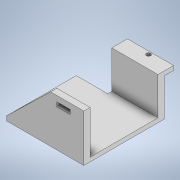
# Autodesk Inventor part: tray2
Saved by Autodesk Inventor 2020 (Build 240168000, 168)
## iProperties
Created: 2022-07-19
Part Number: tray2
Material: 일반
Document SubType Name: Modeling
Designer: SeungJin
Density: 1 g/cm^3
Appearance: 기본값
Author: SeungJin
Autodesk Inventor part; units mm, degrees
ref_plane "YZ Plane" through (0, 0, 0) normal (1, 0, 0) x (0, 1, 0)
ref_plane "XZ Plane" through (0, 0, 0) normal (0, 1, 0) x (-1, 0, 0)
ref_plane "XY Plane" through (0, 0, 0) normal (0, 0, 1) x (1, 0, 0)
sketch "스케치1" plane through (0, 0, 0) normal (0, 1, 0) x (-1, 0, 0)
  line L0 (70.5, 0) -> (70.5, 50)
  line L1 (70.5, 50) -> (0, 50)
  line L2 (0, 50) -> (0, 0)
  line L3 (24.5, 227.5) -> (-40, 227.5)
  line L4 (10, 242.5) -> (37.5, 242.5)
  line L5 (10, 227.5) -> (10, 242.5)
  line L6 (145.5, 227.5) -> (85.5, 227.5)
  line L7 (145.5, 242.5) -> (145.5, 227.5)
  line L8 (85.5, 242.5) -> (145.5, 242.5)
  line L9 (85.5, 227.5) -> (85.5, 242.5)
  line L10 (145.5, 0) -> (145.5, 242.5)
  line L11 (145.5, 242.5) -> (0, 242.5)
  line L12 (0, 242.5) -> (0, 0)
  line L13 (0, 50) -> (145.5, 50)
  circle A0 centre (93.5, 13) radius 2.067
  circle A1 centre (93.5, 37) radius 2.067
  circle A2 centre (147.5, 37) radius 2.067
  circle A3 centre (147.5, 13) radius 2.067
  line L14 (70.5, 0) -> (70.5, 50)
  line L15 (145.5, 50) -> (145.5, 81)
  line L16 (145.5, 75) -> (70.5, 75)
  line L17 (70.5, 50) -> (70.5, 75)
  line L18 (0, 0) -> (0, 25)
  line L19 (145.5, 27.5) -> (0, 27.5)
  line L20 (145.5, 0) -> (145.5, 25)
  line L21 (60.5, 242.5) -> (60.5, 267.5)
  line L22 (60.5, 267.5) -> (27.5, 267.5)
  line L23 (27.5, 267.5) -> (-42.5, 267.5)
  line L24 (145.5, 65) -> (-40, 65)
  circle A4 centre (12.5, 35) radius 2.067
  circle A5 centre (12.5, 15) radius 2.067
  circle A6 centre (-25, 256.5) radius 4.188
  circle A7 centre (12.5, 261) radius 2.067
  circle A8 centre (12.5, 249) radius 2.067
  line L25 (27.5, 242.5) -> (60.5, 242.5)
  line L26 (-40, 242.5) -> (20.5, 242.5)
  line L27 (0, 27.5) -> (0, 65)
  line L28 (145.5, 65) -> (145.5, 27.5)
  line L29 (0, 0) -> (145.5, 0)
  line L30 (24.5, 242.5) -> (24.5, 227.5)
  line L31 (0.5, 227.5) -> (0.5, 242.5)
  line L32 (113.5, 285) -> (113.5, 189)
  line L33 (39.5, 227.5) -> (39.5, 242.5)
  line L34 (39.5, 227.5) -> (24.5, 227.5)
  line L35 (-40, 242.5) -> (-40, 65)
  line L36 (-17.5, 242.5) -> (-17.5, 227.5)
  line L37 (0, 50) -> (-40, 50)
  line L38 (-40, 50) -> (-40, 65)
  point P0 (0, 227.5)
  point P1 (70.5, -15)
  point P2 (85.5, 242.5)
  point P3 (27.5, 242.5)
  point P4 (70.5, 25)
  point P5 (-5, 242.5)
  point P6 (0, 50)
  point P7 (70.5, 65)
  point P8 (0, 50)
  dimension "d1" = 50
  dimension "d3" = 4.134
  dimension "d4" = 4.134
  dimension "d5" = 4.134
  dimension "d6" = 4.134
  dimension "d7" = 12
  dimension "d8" = 12
  dimension "d9" = 32
  dimension "d10" = 15
  dimension "d29" = 40
  dimension "d30" = 30
  constraints: 76 end point, 9 centre point, 9 point on line, 7 vertical, 2 horizontal, 1 midpoint, 1 perpendicular, 14 other
  measures "d1" distance from line of L16 point (70.5, 25)
  measures "d3" diameter of A5
  measures "d4" diameter of A4
  measures "d5" diameter of A8
  measures "d6" diameter of A7
  measures "d7" distance from line of L30 A8.centre
  measures "d8" distance from line of A8.centre L31
  measures "d9" distance between parallel lines of L32 L10
  measures "d10" distance between parallel lines of L33 L30
  measures "d29" distance between parallel lines of L35 L12
  measures "d30" distance from line of L36 A8.centre
extrude "돌출1" add sketch "스케치1" against normal blind 10 contours L1 L12 L24 L17 | L37 L38 L24 L12 | L24 L12 L3 L34 L33 L11 L9 L6 L10 L16 L17 | L24 L35 L3 L12 | L12 L11 L31 L3 | L3 L36 L26 L12 | L31 L11 L5 L3 | L3 L35 L26 L36 | L5 L4 L30 L3 | L6 L32 L8 L7 | L30 L4 L11 L33 L34 | L6 L9 L8 L32
extrude "돌출2" add sketch "스케치1" along normal blind 80 contours L1 L12 L24 L17 | L37 L38 L24 L12 | L12 L11 L31 L3 | L3 L36 L26 L12 | L31 L11 L5 L3 | L3 L35 L26 L36 | L5 L4 L30 L3 | L30 L4 L11 L33 L34
sketch "스케치2" plane through (0, 80, 0) normal (0, 1, 0) x (1, 0, 0)
  line L0 (-39.5, -227.5) -> (-39.5, -242.5) projected
  line L1 (-39.5, -242.5) -> (40, -242.5) projected
  line L2 (40, -227.5) -> (-39.5, -227.5) projected
  line L3 (-39.5, -227.5) -> (40, -227.5) projected
  line L4 (-24.5, -242.5) -> (-0.5, -242.5)
  line L5 (-0.5, -242.5) -> (-0.5, -227.5)
  line L6 (-0.5, -227.5) -> (-24.5, -227.5)
  line L7 (-24.5, -227.5) -> (-24.5, -242.5)
  line L8 (-70.5, -75) -> (-70.5, -50) projected
  line L9 (0, -27.5) -> (-70.5, -27.5)
  line L10 (-70.5, -27.5) -> (-70.5, -65)
  line L11 (40, -242.5) -> (40, -227.5) projected
  line L12 (40, -65) -> (40, -27.5)
  line L13 (40, -65) -> (-70.5, -65) projected
  line L14 (-70.5, -65) -> (40, -65)
  line L15 (40, -27.5) -> (0, -27.5)
  line L16 (7.5, -242.5) -> (7.5, -227.5)
  line L17 (-70.5, -65) -> (40, -65)
  line L18 (40, -65) -> (40, -27.5)
  line L19 (40, -27.5) -> (-70.5, -27.5)
  line L20 (-70.5, -27.5) -> (-70.5, -65)
  point P0 (0, 0)
  point P1 (-0.5, -227.5)
  point P2 (-0.5, -227.5)
  point P3 (-0.5, -242.5)
  point P4 (-12.5, -249)
  point P5 (7.5, -227.5)
  dimension "d15" = 24
  dimension "d16" = 15
  dimension "d31" = 20
  constraints: 28 end point, 5 point on line, 4 parallel, 2 collinear, 2 horizontal, 2 perpendicular, 2 vertical
  measures "d15" distance of L6.end L5.end
  measures "d16" distance between parallel lines of L7 L0
  measures "d31" distance from line of L16 point (-12.5, -249)
extrude "돌출7" add sketch "스케치2" along normal blind 10 contours L2 L7 L1 L0 | L2 L11 L1 L16 | L8 L10 L9 L15 L12 L13
sketch "스케치6" plane through (0, 90, 0) normal (0, 1, 0) x (1, 0, 0)
  line L0 (-39.5, -242.5) -> (-24.5, -242.5) projected
  line L1 (-24.5, -242.5) -> (-24.5, -227.5) projected
  line L2 (-24.5, -227.5) -> (-39.5, -227.5) projected
  line L3 (-39.5, -227.5) -> (-39.5, -242.5) projected
  line L4 (40, -242.5) -> (40, -227.5) projected
  line L5 (40, -227.5) -> (7.5, -227.5) projected
  line L6 (7.5, -227.5) -> (7.5, -242.5) projected
  line L7 (7.5, -242.5) -> (40, -242.5) projected
  line L8 (-39.5, -242.5) -> (40, -242.5)
  line L9 (40, -242.5) -> (40, -227.5)
  line L10 (40, -227.5) -> (-39.5, -227.5)
  line L11 (-39.5, -227.5) -> (-39.5, -242.5)
  point P0 (0, 0)
  constraints: 8 end point, 2 parallel, 1 horizontal, 1 perpendicular
extrude "돌출8" add sketch "스케치6" along normal blind 13
sketch "스케치7" plane through (0, 90, 0) normal (0, 1, 0) x (1, 0, 0)
  point P0 (0, 0)
  point P1 (-12.5, -35)
hole "구멍1" at (-12.5, 90, 35) direction (0, -1, 0) diameter 5.5 end through all counterbore diameter 10 counterbore depth 5 clearance for "Hex Head Cap Screw ISO 24017" size "M5" standard "ISO"
sketch "스케치8" plane through (0, 0, 0) normal (0, 1, 0) x (1, 0, 0)
  line L0 (-145.5, -75) -> (-145.5, -242.5) projected
  line L1 (-39.5, -227.5) -> (40, -227.5) projected
  line L2 (-145.5, -242.5) -> (-39.5, -242.5)
  line L3 (-39.5, -242.5) -> (-39.5, -227.5)
  line L4 (-39.5, -227.5) -> (-145.5, -227.5)
  line L5 (-145.5, -227.5) -> (-145.5, -242.5)
  point P0 (0, 0)
  constraints: 8 end point, 2 parallel, 1 horizontal, 1 perpendicular
extrude "돌출9" add sketch "스케치8" along normal up to surface (103 mm away)
sketch "스케치9" plane through (-145.5, -10, 242.5) normal (0, 0, 1) x (1, 0, 0)
  line L0 (153, 90) -> (153, 100) projected
  line L1 (121, 90) -> (153, 90) projected
  line L2 (121, 90) -> (121, 100) projected
  line L3 (121, 100) -> (153, 100) projected
  line L4 (185.5, 0) -> (185.5, 113) projected
  line L5 (185.5, 113) -> (0, 113) projected
  line L6 (0, 113) -> (0, 0) projected
  line L7 (185.5, 0) -> (0, 0) projected
  line L8 (106, 113) -> (106, 0)
  line L9 (75, 0) -> (185.5, 0) projected
  line L10 (75, 10) -> (0, 10) projected
  line L11 (106, 113) -> (0, 10)
  point P0 (145.5, 10)
  dimension "d45" = 79.5
  constraints: 4 end point, 2 point on line, 1 vertical
  measures "d45" distance between parallel lines of L4 L8
extrude "돌출10" cut sketch "스케치9" against normal up to surface (15 mm away) contours L11 L6 L5
